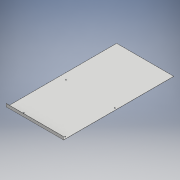
# Autodesk Inventor part: my trunk
Saved by Autodesk Inventor 2018 (Build 220112000, 112)
## iProperties
Created: 2018-06-19
Part Number: my trunk
Material: Generic
Document SubType Name: Sheet Metal
Designer: John Viljoen
Density: 1 g/cm^3
Sheet Metal Rule: Default_mm
Appearance: Default
Author: John Viljoen
Autodesk Inventor part; units mm, degrees
ref_plane "YZ Plane" through (0, 0, 0) normal (1, 0, 0) x (0, 1, 0)
ref_plane "XZ Plane" through (0, 0, 0) normal (0, 1, 0) x (-1, 0, 0)
ref_plane "XY Plane" through (0, 0, 0) normal (0, 0, 1) x (1, 0, 0)
sketch "Sketch1" plane through (0, 0, 0) normal (0, 0, 1) x (1, 0, 0)
  line L0 (0, 0) -> (181.174, 0)
  line L1 (181.174, 0) -> (181.174, 350.17)
  line L2 (181.174, 350.17) -> (0, 350.17)
  line L3 (0, 350.17) -> (0, 0)
  dimension "d0" = 181.174
  dimension "d1" = 350.17
  measures "d0" distance of L2.end L1.end
  measures "d1" distance of L1.end L0.end
extrude "Plate1" add sketch "Sketch1" along normal blind 0.5
sketch "Sketch2" plane through (0, 0, 0.5) normal (0, 0, 1) x (1, 0, 0)
  line L0 (181.174, 350.17) -> (181.174, 0) projected
  line L1 (181.174, 0) -> (181.174, 350.17) construction
  line L2 (181.174, 164.4082) -> (174.824, 164.4082) construction
  line L3 (174.824, 164.4082) -> (174.824, 169.4082) construction
  line L4 (181.174, 6.9282) -> (174.824, 6.9282) construction
  line L5 (174.824, 6.9282) -> (174.824, 11.9282) construction
  line L6 (174.824, 11.9282) -> (42.744, 11.9282) construction
  line L7 (174.824, 169.4082) -> (19.884, 169.4082) construction
  circle A0 centre (19.884, 169.4082) radius 1.5
  circle A1 centre (174.824, 169.4082) radius 1.5
  circle A2 centre (174.824, 11.9282) radius 1.5
  circle A3 centre (43.5456, 11.9282) radius 1.5
  point P0 (83.2182, 85.7582)
  dimension "d3" = 6.35
  dimension "d4" = 5
  dimension "d5" = 6.35
  dimension "d6" = 5
  dimension "d8" = 132.08
  dimension "d9" = 154.94
  dimension "d10" = 3
  dimension "d11" = 3
  dimension "d12" = 3
  dimension "d13" = 3
  constraints: 12 end point, 4 centre point, 4 perpendicular, 3 coincident, 3 point on line, 2 horizontal
  measures "d3" distance of L2.start L2.end
  measures "d4" distance of L2.end L3.end
  measures "d5" distance of L4.start L4.end
  measures "d6" distance of L4.end L5.end
  measures "d8" distance of L5.end L6.end
  measures "d9" distance of L3.end L7.end
  measures "d10" diameter of A0
  measures "d11" diameter of A1
  measures "d12" diameter of A2
  measures "d13" diameter of A3
extrude "Extrusion1" cut sketch "Sketch2" against normal blind 10
sketch "Sketch3" plane through (181.174, 0.5, 0) normal (0, -1, 0) x (1, 0, 0)
  line L0 (-181.174, 0) -> (0, 0)
  line L1 (0, 0) -> (0, 10)
  line L2 (0, 10) -> (-181.174, 10)
  line L3 (-181.174, 10) -> (-181.174, 0)
  constraints: 6 end point, 1 horizontal, 1 perpendicular, 1 vertical
edge flange "Flange1" height 10 angle 90 thickness 0.5 bend radius 0.5 thickness toward (0, -1, 0) relief straight relief width 0.5 relief depth 0.25 edges at (90.587, 0, 0.5) wall of the first edge with corners at (0, 0.5, 0) (181.174, 0.5, 0) (181.174, 0.5, 10) (0, 0.5, 10)
bend "Bend1"
corner "Corner1"
equation "\"d2\" = Thickness"
equation "\"d16\" = BendReliefWidth"
equation "\"d17\" = BendReliefDepth"
equation "\"d18\" = MinimumRemnant"
equation "\"d19\" = TransitionRadius"
equation "\"d22\" = BendRadius"
equation "\"d23\" = CornerReliefSize"
equation "\"d24\" = GapSize"
equation "\"d25\" = JacobiRadiusSize"
equation "\"BendRadius\" = Thickness"
equation "\"BendReliefWidth\" = Thickness"
equation "\"BendReliefDepth\" = 0.5 * Thickness"
equation "\"CornerReliefSize\" = 4 * Thickness"
equation "\"MinimumRemnant\" = 2 * Thickness"
equation "\"TransitionRadius\" = BendRadius"
equation "\"JacobiRadiusSize\" = BendRadius"
equation "\"GapSize\" = Thickness"
equation "\"Thickness\" = 0.5"
body "Solid1"
